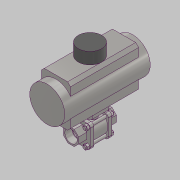
# Autodesk Inventor part: PNEUMATIC THREADED BALL VALVE DN15 S235
Saved by Autodesk Inventor 2017 (Build 210142000, 142)
## iProperties
Category: Plant Design Equipment
Company: Pocket Brewery Belgium
Created: 2017-11-25
Part Number: PNEUMATIC THREADED BALL VALVE DN15 S235
Material: S235
Document SubType Name: Modeling
Designer: Demarec
Density: 7.85 g/cm^3
Appearance: Semi-Polished
Description: BELVEN BV3
Author: Marc Crauwels
Title: Valves
Comments: This Valve is generated with the Pocket Brewery Valve App. This software is part of the Pocket Brewery Design Suite.
Autodesk Inventor part; units mm, degrees
ref_plane "YZ Plane" through (0, 0, 0) normal (1, 0, 0) x (0, 1, 0)
ref_plane "XZ Plane" through (0, 0, 0) normal (0, 1, 0) x (-1, 0, 0)
sketch "Sketch3" plane through (0, 0, 0) normal (0, 1, 0) x (-1, 0, 0)
  line L0 (-5.3576, 12.9343) -> (5.3576, 12.9343)
  line L1 (5.3576, 12.9343) -> (12.9343, 5.3576)
  line L2 (12.9343, 5.3576) -> (12.9343, -5.3576)
  line L3 (12.9343, -5.3576) -> (5.3576, -12.9343)
  line L4 (5.3576, -12.9343) -> (-5.3576, -12.9343)
  line L5 (-5.3576, -12.9343) -> (-12.9343, -5.3576)
  line L6 (-12.9343, -5.3576) -> (-12.9343, 5.3576)
  line L7 (-12.9343, 5.3576) -> (-5.3576, 12.9343)
  circle A0 centre (0, 0) radius 14
  line L8 (14.25, -19) -> (-14.25, -19)
  line L9 (-19, -14.25) -> (-19, 14.25)
  line L10 (-14.25, 19) -> (14.25, 19)
  line L11 (19, 14.25) -> (19, -14.25)
  line L12 (19, -19) -> (-19, 19) construction
  line L13 (-19, -19) -> (19, 19) construction
  circle A1 centre (0, 0) radius 12.9343
  arc A2 (19, 14.25) -> (14.25, 19) centre (14.25, 14.25) ccw
  arc A3 (-14.25, 19) -> (-19, 14.25) centre (-14.25, 14.25) ccw
  arc A4 (-19, -14.25) -> (-14.25, -19) centre (-14.25, -14.25) ccw
  arc A5 (14.25, -19) -> (19, -14.25) centre (14.25, -14.25) ccw
  circle A6 centre (0, 0) radius 10.65
  circle A7 centre (14.25, 14.25) radius 2.5
  circle A8 centre (0, 0) radius 18
  circle A9 centre (0, 0) radius 9.15
  dimension "d72" = 28
  dimension "oFlangeW" = 38
  dimension "d2" = 4.75
  dimension "oIntDia" = 21.3
  dimension "oMbolt" = 5
  dimension "d16" = 4
  dimension "d73" = 1.5
  constraints: 28 end point, 9 centre point, 9 tangent, 8 point on circle, 8 point on line, 5 coincident, 3 equal radius, 2 horizontal, 2 midpoint, 2 parallel, 2 perpendicular, 20 other
  measures "oFlangeW" distance of L12.start L13.start
  measures "d2" radius of A2
  measures "oIntDia" diameter of A6
  measures "oMbolt" diameter of A7
  measures "d73" radial gap between concentric circles of A6 A9
extrude "Extrusion1" add sketch "Sketch3" along normal mid plane 65 contours L0 A1 L7 | L0 L1 A1 | A1 | A1 L6 L7 | L1 L2 A1 | A1 L5 L6 | L2 L3 A1 | A1 L4 L5 | L3 L4 A1
extrude "Extrusion2" add sketch "Sketch3" along normal mid plane 37 contours A0 L0 | L7 A0 | A0 L1 | L6 A0 | A0 L2 | L5 A0 | L4 A0 | A0 L3 | L8 A4 L9 A3 L10 A2 L11 A5 | A7 A8 | A8 A7 | A7 A8
extrude "Extrusion3" cut sketch "Sketch3" along normal mid plane 25 contours L8 A4 L9 A3 L10 A2 L11 A5 | A7 A8 picked at (13.8519, 13.7915)
extrude "Extrusion4" add sketch "Sketch3" along normal mid plane 48 contours A7 A8 | A8 A7 picked at (13.8519, 13.7915) picked at (12.5879, 12.7058)
sketch "Sketch4" plane through (0, -18.5, 0) normal (0, -1, 0) x (1, 0, 0)
  circle A0 centre (-14.25, 14.25) radius 2.5 projected
  line L0 (-12.0849, 10.5) -> (-16.4151, 10.5)
  line L1 (-16.4151, 10.5) -> (-18.5801, 14.25)
  line L2 (-18.5801, 14.25) -> (-16.4151, 18)
  line L3 (-16.4151, 18) -> (-12.0849, 18)
  line L4 (-12.0849, 18) -> (-9.9199, 14.25)
  line L5 (-9.9199, 14.25) -> (-12.0849, 10.5)
  point P0 (0, 0)
  dimension "d13" = 7.5
  constraints: 12 end point, 1 coincident, 1 horizontal, 13 other
  measures "d13" distance between parallel lines of L0 L3
extrude "Extrusion5" add sketch "Sketch4" along normal blind 4
mirror "Mirror1" about plane through (0, 0, 0) normal (0, 1, 0) of "Extrusion5"
pattern_circular "Circular Pattern1" count 4 over 360 about axis through (0, 0, 0) along (0, 1, 0) of "Extrusion5", "Extrusion4", "Mirror1"
ref_plane "Work Plane1" through (0, 0, 32) normal (0, 0, 1) x (1, 0, 0)
sketch "Sketch5" plane through (0, 0, 32) normal (0, 0, 1) x (1, 0, 0)
  line L0 (-13.25, -18) -> (13.25, -18)
  line L1 (18, -13.25) -> (18, 13.25)
  line L2 (13.25, 18) -> (-13.25, 18)
  line L3 (-18, 13.25) -> (-18, -13.25)
  line L4 (-18, -18) -> (18, 18) construction
  line L5 (18, -18) -> (-18, 18) construction
  arc A0 (-18, -13.25) -> (-13.25, -18) centre (-13.25, -13.25) ccw
  arc A1 (13.25, -18) -> (18, -13.25) centre (13.25, -13.25) ccw
  arc A2 (18, 13.25) -> (13.25, 18) centre (13.25, 13.25) ccw
  arc A3 (-13.25, 18) -> (-18, 13.25) centre (-13.25, 13.25) ccw
  point P0 (0, 0)
  dimension "d21" = 36
  dimension "d22" = 4.75
  constraints: 12 end point, 8 point on circle, 8 point on line, 8 tangent, 4 centre point, 3 equal radius, 2 midpoint, 2 parallel, 2 perpendicular, 1 horizontal
  measures "d21" distance of L4.start L5.start
  measures "d22" radius of A0
extrude "Extrusion6" add sketch "Sketch5" against normal blind 7
sketch "Sketch6" plane through (0, 0, 25) normal (0, 0, -1) x (-1, 0, 0)
  circle A0 centre (0, 0) radius 10.65
  dimension "d25" = 21.3
  constraints: 1 centre point, 1 coincident
  measures "d25" diameter of A0
extrude "Extrusion7" add sketch "Sketch6" along normal up to surface
sketch "Sketch11" plane through (0, 0, 0) normal (0, 1, 0) x (-1, 0, 0)
  line L0 (25, 32) -> (-25, 32)
  line L1 (-25, 32) -> (-25, 104)
  line L2 (-25, 104) -> (25, 104)
  line L3 (25, 104) -> (25, 32)
  line L4 (-25, 104) -> (25, 32) construction
  line L5 (25, 104) -> (-25, 32) construction
  circle A0 centre (0, 68) radius 30
  line L6 (0, 104) -> (-20, 104)
  line L7 (-20, 104) -> (-20, 124)
  line L8 (-20, 124) -> (0, 124)
  line L9 (0, 124) -> (0, 104)
  circle A1 centre (0, 0) radius 18 projected
  line L10 (0, 0) -> (0, 68)
  line L11 (-13.25, 32) -> (13.25, 32) projected
  dimension "oCylinderWeight" = 50
  dimension "oCylinderHeight" = 72
  dimension "oCylinderDia" = 60
  dimension "d62" = 20
  dimension "d63" = 20
  constraints: 22 end point, 4 parallel, 2 horizontal, 2 midpoint, 2 perpendicular, 1 centre point, 1 collinear, 1 vertical
  measures "oCylinderWeight" distance of L1.end L2.end
  measures "oCylinderHeight" distance of L0.end L1.end
  measures "oCylinderDia" diameter of A0
  measures "d62" distance of L7.end L8.end
  measures "d63" distance of L6.end L7.end
extrude "Extrusion12" add sketch "Sketch11" along normal mid plane 147 contours A0 L1 L3 | L3 A0 | L1 A0
extrude "Extrusion13" add sketch "Sketch11" along normal mid plane 117 contours L0 L10 A0 L3 | A0 L1 L3 | L0 L1 A0 L10 | A0 L1 L2 L3
revolve "Revolution1" add sketch "Sketch11" angle 360 about axis through (0, 0, 124) along (0, 0, -1) contours L2 L7 L8 L9
chamfer "Chamfer3" distance 5 angle 45 4 edges at (25, 0, 104) (-25, 0, 104) (-25, 0, 32) (25, 0, 32)
extrude "Extrusion14" add sketch "Sketch3" along normal mid plane 41 contours A6
equation "\"d2\" = 0.125 * oFlangeW"
equation "\"d13\" = 1.5 * oMbolt"
equation "\"d14\" = 0.8 * oMbolt"
equation "\"d22\" = d2"
equation "\"d25\" = oIntDia"
body "Solid1"
